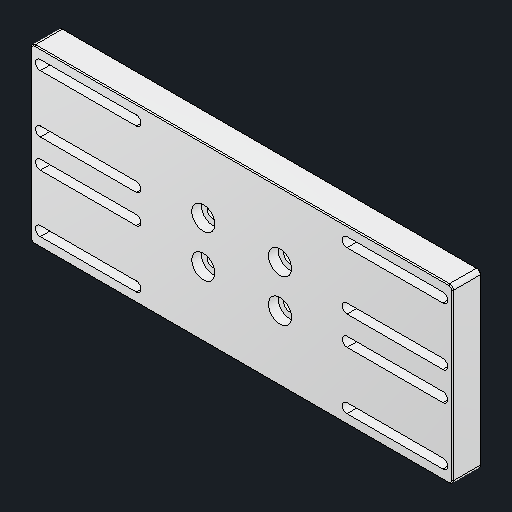
# Autodesk Inventor part: clamp-foot-double
Saved by Autodesk Inventor 2027.1 (Build 311270010, 270A)
## iProperties
Created: 2026-10-07
Part Number: clamp-foot-double
Material: Aluminum 6061
Document SubType Name: Modeling
Designer: queezz
Density: 2.7 g/cm^3
Appearance: Aluminum - Flat
Mass: 704.823 g
Surface Area: 593.324 cm^2
Volume: 261.046 cm^3
Author: queezz
Autodesk Inventor part; units mm, degrees
ref_plane "YZ Plane" through (0, 0, 0) normal (1, 0, 0) x (0, 1, 0)
ref_plane "XY Plane" through (0, 0, 0) normal (0, 0, 1) x (1, 0, 0)
sketch "Sketch1" plane through (0, 0, 0) normal (0, 0, 1) x (1, 0, 0)
  line L0 (-110, 22.5) -> (110, 22.5)
  line L1 (110, 22.5) -> (110, -22.5)
  line L2 (110, -22.5) -> (-110, -22.5)
  line L3 (-110, -22.5) -> (-110, 22.5)
  point P0 (0, 0)
  point P1 (110, 0)
  point P2 (0, 22.5)
  dimension "d0" = 220
  dimension "d1" = 45
  constraints: 8 end point, 2 midpoint, 2 parallel, 1 horizontal, 1 horizontal alignment, 1 perpendicular, 1 vertical alignment
  measures "d0" distance of L0.start L0.end
  measures "d1" distance of L0.end L1.end
extrude "Extrusion1" add sketch "Sketch1" along normal blind 15
sketch "Sketch2" plane through (0, 0, 15) normal (0, 0, 1) x (1, 0, 0)
  line L0 (-105, 15) -> (-55, 15) construction
  line L1 (-105, 12.5) -> (-55, 12.5)
  line L2 (-55, 17.5) -> (-105, 17.5)
  arc A0 (-105, 17.5) -> (-105, 12.5) centre (-105, 15) ccw
  arc A1 (-55, 12.5) -> (-55, 17.5) centre (-55, 15) ccw
  line L3 (-105, -15) -> (-55, -15) construction
  line L4 (-105, -17.5) -> (-55, -17.5)
  line L5 (-55, -12.5) -> (-105, -12.5)
  arc A2 (-105, -12.5) -> (-105, -17.5) centre (-105, -15) ccw
  arc A3 (-55, -17.5) -> (-55, -12.5) centre (-55, -15) ccw
  line L6 (-80, 15) -> (-80, -15) construction
  line L7 (-110, 22.5) -> (-110, -22.5) projected
  point P0 (0, 0)
  point P1 (-80, 0)
  dimension "d4" = 5
  dimension "d5" = 30
  dimension "d6" = 50
  dimension "d7" = 5
  constraints: 18 end point, 8 point on circle, 8 tangent, 4 centre point, 4 parallel, 3 midpoint, 1 equal radius, 1 horizontal, 1 horizontal alignment, 1 vertical
  measures "d4" diameter of A1
  measures "d5" distance between parallel lines of L3 L0
  measures "d6" distance of L2.start L2.end
  measures "d7" distance from line of L7 L0.start
extrude "Extrusion2" cut sketch "Sketch2" against normal through all
mirror "Mirror1" about plane through (0, 0, 0) normal (1, 0, 0) of "Extrusion2"
fillet "Fillet1" [suppressed]
chamfer "Chamfer1" [suppressed]
sketch "Sketch3" plane through (0, 0, 15) normal (0, 0, -1) x (-1, 0, 0)
  line L0 (-20, -11.5) -> (20, -11.5) construction
  line L1 (-110, 22.5) -> (110, 22.5) projected
  line L2 (110, -22.5) -> (-110, -22.5) projected
  point P0 (0, 0)
  point P1 (0, -11.5)
  dimension "d14" = 40
  dimension "d28" = 11
  constraints: 2 coincident, 2 end point, 1 horizontal, 1 midpoint, 1 vertical alignment
  measures "d14" distance of L0.start L0.end
  measures "d28" distance between parallel lines of L2 L0
hole "Hole1" at (20, -11.5, 15) at (-20, -11.5, 15) direction (0, 0, -1) diameter 6 end through all counterbore diameter 12 counterbore depth 5
ref_plane "Middle joining plane" through (0, -22.5, 0) normal (0, 1, 0) x (-1, 0, 0)
mirror "Double short side - join solid" about plane through (0, -22.5, 0) normal (0, 1, 0)
fillet "Double plate outer corners - R2" radius 2 4 edges at (110, -67.5, 7.5) (-110, -67.5, 7.5) (-110, 22.5, 7.5) (110, 22.5, 7.5)
chamfer "Double plate perimeter - 0.5 mm chamfer" distance 0.5 angle 45 12 edges at (109.4142, 21.9142, 15) (0, 22.5, 15) (-109.4142, 21.9142, 15) (-110, -22.5, 15) (0, -67.5, 15) (110, -22.5, 15) (109.4142, 21.9142, 0) (110, -22.5, 0) (0, -67.5, 0) (-110, -22.5, 0) (-109.4142, 21.9142, 0) (0, 22.5, 0)
equation "\"d28\" = bolts"
equation "\"bolts\" = 11"
body "Solid1"
